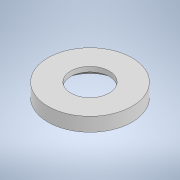
# Autodesk Inventor part: Корпус сальника
Saved by Autodesk Inventor 2021 (Build 250183000, 183)
## iProperties
Created: 2020-11-05
Part Number: Корпус сальника
Material: Типовые
Document SubType Name: Modeling
Designer: Тимоха
Density: 1 g/cm^3
Appearance: По умолчанию
Author: Тимоха
Autodesk Inventor part; units mm, degrees
ref_plane "YZ Plane" through (0, 0, 0) normal (1, 0, 0) x (0, 1, 0)
ref_plane "XZ Plane" through (0, 0, 0) normal (0, 1, 0) x (-1, 0, 0)
ref_plane "XY Plane" through (0, 0, 0) normal (0, 0, 1) x (1, 0, 0)
sketch "Эскиз1" plane through (0, 0, 0) normal (0, 0, 1) x (1, 0, 0)
  line L0 (0, 0) -> (0, 20)
  line L1 (70, 0) -> (50, 0)
  line L2 (50, 0) -> (50, 15)
  line L3 (32, 20) -> (32, 15)
  line L4 (32, 15) -> (32, 23)
  line L5 (32, 23) -> (70, 23)
  line L6 (70, 0) -> (70, 23)
  line L7 (32, 15) -> (50, 15)
  dimension "d2" = 20
  dimension "d3" = 15
  dimension "d4" = 32
  dimension "d6" = 8
  constraints: 16 end point, 2 vertical, 1 horizontal, 1 perpendicular, 1 point on line
  measures "d2" distance of L1.start L1.end
  measures "d3" distance of L1.end L2.end
  measures "d4" distance of L0.end L3.start
  measures "d6" distance of L3.end L4.end
revolve "Вращение1" add sketch "Эскиз1" angle 360 about axis through (0, 0, 0) along (0, 1, 0)
